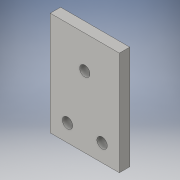
# Autodesk Inventor part: limit-holders_CPY
Saved by Autodesk Inventor 2016 (Build 200138000, 138)
## iProperties
Created: 2018-04-04
Part Number: limit-holders_CPY
Material: Generic
Document SubType Name: Modeling
Designer: Nuwan
Density: 1 g/cm^3
Appearance: Default
Author: Nuwan
Autodesk Inventor part; units mm, degrees
ref_plane "YZ Plane" through (0, 0, 0) normal (1, 0, 0) x (0, 1, 0)
ref_plane "XZ Plane" through (0, 0, 0) normal (0, 1, 0) x (-1, 0, 0)
ref_plane "XY Plane" through (0, 0, 0) normal (0, 0, 1) x (1, 0, 0)
sketch "Sketch1" plane through (0, 0, 0) normal (0, 0, 1) x (1, 0, 0)
  line L0 (0, 0) -> (20, 0)
  line L1 (20, 0) -> (20, 30)
  line L2 (20, 30) -> (0, 30)
  line L3 (0, 30) -> (0, 0)
  dimension "d0" = 20
  dimension "d1" = 30
  constraints: 8 end point, 2 parallel, 1 horizontal, 1 perpendicular
  measures "d0" distance of L2.end L1.end
  measures "d1" distance of L1.end L0.end
extrude "Extrusion1" add sketch "Sketch1" along normal blind 3
sketch "Sketch2" plane through (0, 0, 3) normal (0, 0, 1) x (1, 0, 0)
  line L0 (0, 0) -> (20, 0) projected
  line L1 (20, 0) -> (20, 30) projected
  line L2 (20, 30) -> (0, 30) projected
  line L3 (0, 30) -> (0, 0) projected
  line L4 (0, 5) -> (20, 5)
  line L5 (10, 0) -> (10, 30)
  circle A0 centre (5, 5) radius 1.5
  circle A1 centre (15, 5) radius 1.5
  dimension "d4" = 3
  dimension "d5" = 10
  dimension "d6" = 10
  constraints: 4 end point, 3 point on line, 2 centre point, 2 midpoint, 1 perpendicular, 1 symmetric about line, 1 other
  measures "d4" diameter of A0
  measures "d5" diameter of A0.centre L5
  measures "d6" diameter of L0 L4
extrude "Extrusion2" cut sketch "Sketch2" against normal blind 3 contours A0 L4 | L4 A0 | A1 L4 | L4 A1
sketch "Sketch4" plane through (0, 0, 3) normal (0, 0, 1) x (1, 0, 0)
  line L0 (0, 0) -> (20, 0) projected
  line L1 (20, 30) -> (0, 30) projected
  line L2 (10, 30) -> (10, 0)
  circle A0 centre (10, 20.5) radius 1.5
  dimension "d13" = 3
  dimension "d14" = 9.5
  constraints: 2 end point, 2 midpoint, 1 centre point, 1 point on line
  measures "d13" diameter of A0
  measures "d14" distance from line of L1 A0.centre
extrude "Extrusion4" cut sketch "Sketch4" against normal blind 3
body "Solid1"
